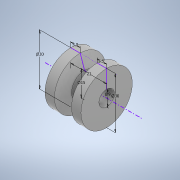
# Autodesk Inventor part: Pulley
Saved by Autodesk Inventor 2020 (Build 240168000, 168)
## iProperties
Created: 2021-12-06
Part Number: Pulley
Material: ABS Plastic
Document SubType Name: Modeling
Designer: Umur Batuhan Özmen
Density: 1.06 g/cm^3
Appearance: Smooth - Medium Gray
Author: Umur Batuhan Özmen
Autodesk Inventor part; units mm, degrees
ref_plane "YZ Plane" through (0, 0, 0) normal (1, 0, 0) x (0, 1, 0)
ref_plane "XZ Plane" through (0, 0, 0) normal (0, 1, 0) x (-1, 0, 0)
ref_plane "XY Plane" through (0, 0, 0) normal (0, 0, 1) x (1, 0, 0)
sketch "Sketch1" plane through (0, 0, 0) normal (0, 0, 1) x (1, 0, 0)
  line L0 (10.5, 24.5) -> (-10.5, 24.5)
  line L1 (-10.5, 24.5) -> (-10.5, 35)
  line L2 (10.5, 24.5) -> (10.5, 35)
  line L3 (-10.5, 35) -> (-5, 35)
  line L4 (10.5, 35) -> (5, 35)
  line L5 (2.4732, 27.5) -> (-2.4732, 27.5)
  line L6 (-5, 35) -> (6.4911, 35) construction
  line L7 (5, 35) -> (16.4911, 35) construction
  line L8 (-25.5367, 20) -> (30.733, 20)
  line L9 (-5, 35) -> (-2.4732, 27.5)
  line L10 (2.4732, 27.5) -> (5, 35)
  point P0 (0, 0)
  dimension "d2" = 21
  dimension "d4" = 5.5
  dimension "d5" = 5.5
  dimension "d44" = 9
  dimension "d48" = 15
  dimension "d49" = 30
  dimension "d50" = 30
  constraints: 22 end point, 6 horizontal, 2 vertical
  measures "d2" distance of L0.start L0.end
  measures "d4" distance of L1.end L3.end
  measures "d5" distance of L2.end L4.end
  measures "d44" diameter of L0 L8
  measures "d48" diameter of L5 L8
  measures "d49" diameter of L3 L8
  measures "d50" diameter of L4 L8
revolve "Revolution1" add sketch "Sketch1" angle 360 about axis through (-25.5367, 20, 0) along (1, 0, 0)
body "Solid1"
